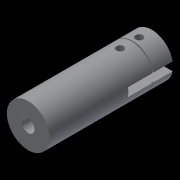
# Autodesk Inventor part: PelvisMountStem
Saved by Autodesk Inventor 2015 (Build 190159000, 159)
## iProperties
RuleStatus: InUse
Created: 2014-12-11
Part Number: PelvisMountStem
Material: Generic
Document SubType Name: Modeling
Designer: Inventor
Mass: 15.5644 g
Surface Area: 59.1598 cm^2
Volume: 15.5644 cm^3
Density: 1 g/cm^3
Appearance: Default
BeforeDocSave0: UpdateBoundingBox
CX: 20.00 mm
CY: 58.00 mm
CZ: 20.00 mm
Author: Inventor
Autodesk Inventor part; units mm, degrees
ref_plane "YZ Plane" through (0, 0, 0) normal (1, 0, 0) x (0, 1, 0)
ref_plane "XZ Plane" through (0, 0, 0) normal (0, 1, 0) x (-1, 0, 0)
sketch "Body" plane through (0, 0, 0) normal (0, 0, 1) x (1, 0, 0)
  circle A0 centre (0, 0) radius 1.75
  line L0 (-10, -52) -> (10, -52)
  line L1 (10, 6) -> (-10, 6)
  line L2 (10, 6) -> (10, -52)
  line L3 (-10, 6) -> (-10, -52)
  line L4 (0, -52) -> (0, 6)
  line L5 (10, -15) -> (-10, -15)
  circle A1 centre (0, -9) radius 1.75
  circle A2 centre (0, 0) radius 2.75 construction
  circle A3 centre (0, -9) radius 2.75 construction
  line L6 (-7.5, 6) -> (-7.5, -15)
  dimension "d0" = 58
  dimension "d2" = 3.5
  dimension "d3" = 6
  dimension "d5" = 10
  dimension "d6" = 20
  dimension "d7" = 9
  dimension "d23" = 5.5
  dimension "d25" = 6
  dimension "d26" = 2.5
  constraints: 14 end point, 6 point on line, 4 centre point, 3 coincident, 2 equal radius, 2 midpoint, 2 perpendicular, 2 vertical, 1 horizontal
  measures "d0" distance of L1.end L3.end
  measures "d2" diameter of A0
  measures "d3" distance from line of L1 A0.centre
  measures "d5" distance between parallel lines of L2 L4
  measures "d6" distance of L3.end L2.end
  measures "d7" distance of A1.centre A0.centre
  measures "d23" diameter of A2
  measures "d25" distance from line of L5 A1.centre
  measures "d26" distance between parallel lines of L6 L3
revolve "BodyFeature" add sketch "Body" angle 360 about axis through (0, -52, 0) along (0, 1, 0) picked at (-0.4801, -0.3314) picked at (-0.4801, -8.6686) contours L4 A0 | A0 L4 A1 L5 L6 L1 | L4 A1 | L6 L5 L3 L1 | L5 L4 L0 L3
extrude "HolesFeature" cut sketch "Body" along normal through all both and the other way through all contours A0 L4 | L4 A0 | A1 L4 | L4 A1
extrude "MountFeature" cut sketch "Body" along normal mid plane 4 contours A0 L4 L1 L2 L5 A1 | A0 L4 A1 L5 L6 L1
ref_plane "TopGroovePlane" through (-7.5, -3, -2) normal (0, 1, 0) x (1, 0, 0)
sketch "TopGroove" plane through (-7.5, -3, -2) normal (0, 1, 0) x (1, 0, 0)
  circle A0 centre (7.5, -2) radius 10 projected
  circle A1 centre (7.5, -2) radius 9.3
  dimension "d30" = 0.7
  constraints: 1 centre point, 1 coincident
  measures "d30" radial gap between concentric circles of A0 A1
extrude "TopGrooveFeature" cut sketch "TopGroove" against normal blind 0.5
sketch "BottomMountHole" plane through (0, -52, 0) normal (0, -1, 0) x (1, 0, 0)
  circle A0 centre (0, 0) radius 10 projected
hole "BottomMountHoleFeature" at (0, -52, 0) direction (0, 1, 0) diameter 6 depth 30 tip angle 118
